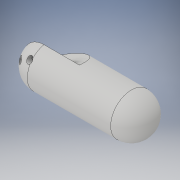
# Autodesk Inventor part: P1704_003_mainGauche
Saved by Autodesk Inventor 2019 (Build 230136000, 136)
## iProperties
Created: 2019-04-29
Part Number: P1704_003_mainGauche
Material: Générique
Document SubType Name: Modeling
Designer: Joan.MAILLARD
Density: 1 g/cm^3
Appearance: Par défaut
Author: Joan.MAILLARD
Autodesk Inventor part; units mm, degrees
ref_plane "YZ Plane" through (0, 0, 0) normal (1, 0, 0) x (0, 1, 0)
ref_plane "XZ Plane" through (0, 0, 0) normal (0, 1, 0) x (-1, 0, 0)
sketch "Esquisse1" plane through (0, 0, 0) normal (0, 1, 0) x (-1, 0, 0)
  line L0 (0, 0) -> (-100, 0)
  line L1 (-100, 0) -> (-100, -25)
  line L2 (-100, -25) -> (0, -25)
  line L3 (0, -25) -> (0, 0)
  arc A0 (0, -25) -> (25, 0) centre (0, 0) ccw
  line L4 (25, 0) -> (0, 0)
  line L5 (0, 0) -> (0, -25)
  line L6 (-100, 0) -> (-100, -25)
  arc A1 (-125, 0) -> (-100, -25) centre (-100, 0) ccw
  line L7 (-100, 0) -> (-125, 0)
  dimension "d1" = 25
  dimension "d2" = 100
  constraints: 16 end point, 4 line through centre, 4 point on circle, 3 equal length, 2 centre point, 2 coincident, 2 horizontal, 2 perpendicular, 1 vertical
  measures "d1" distance of L2.end L0.start
  measures "d2" distance of L1.end L2.end
revolve "Révolution1" add sketch "Esquisse1" angle 360 about axis through (0, 0, 0) along (1, 0, 0)
ref_plane "Plan de construction1" through (50, 0, -25) normal (0, 0, 1) x (1, 0, 0)
sketch "Esquisse2" plane through (50, 0, -25) normal (0, 0, 1) x (1, 0, 0)
  arc A0 (-50, 25) -> (-50, -25) centre (-50, 0) ccw projected
  line L0 (-50, 0) -> (-71.6506, -12.5)
  line L1 (-71.6506, -12.5) -> (-84.1506, 9.1506)
  line L2 (-84.1506, 9.1506) -> (-62.5, 21.6506)
  line L3 (-62.5, 21.6506) -> (-50, 0)
  line L4 (-50, 0) -> (-31.3481, 0) construction
  line L5 (-50, 0) -> (-62.5, 21.6506)
  line L6 (-62.5, 21.6506) -> (-19.1987, 46.6506)
  line L7 (-19.1987, 46.6506) -> (-6.6987, 25)
  line L8 (-6.6987, 25) -> (-50, 0)
  line L9 (-50, -25) -> (-50, 25) construction
  line L10 (-50, 25) -> (75, 25) construction
  line L11 (-50, 25) -> (50, 25) construction
  dimension "d9" = 120
  constraints: 20 end point, 4 parallel, 3 perpendicular, 2 point on circle, 2 point on line, 1 horizontal
  measures "d9" angle of L4 L3
extrude "Extrusion1" cut sketch "Esquisse2" along normal blind 30
ref_plane "Plan de construction2" through (50, 0, 35) normal (0, 0, -1) x (-1, 0, 0)
sketch "Esquisse3" plane through (50, 0, 35) normal (0, 0, -1) x (-1, 0, 0)
  line L0 (50, 0) -> (71.2132, -12.2474) construction
  line L1 (71.2132, -12.2474) -> (50, 0) construction
  line L2 (50, 0) -> (50, 0) construction
  line L3 (65.2228, 7.3769) -> (52.2324, 14.8769) construction
  circle A0 centre (65.2228, 7.3769) radius 1.7
  circle A1 centre (52.2324, 14.8769) radius 1.7
  line L4 (71.2132, -12.2474) -> (93.5005, 26.3552) construction
  line L5 (52.2324, 14.8769) -> (45.2324, 2.7526) construction
  line L6 (6.6987, 25) -> (-50, 25) construction
  dimension "d12" = 14
  dimension "d22" = 3.4
  dimension "d23" = 3.4
  dimension "d30" = 15
  dimension "d31" = 30
  constraints: 8 end point, 2 centre point, 2 coincident, 2 perpendicular, 1 collinear, 1 parallel, 1 other
  measures "d12" distance from line of L0 L3.start
  measures "d22" diameter of A0
  measures "d23" diameter of A1
  measures "d30" distance from line of L4 A0.centre
  measures "d31" distance from line of L4 L5.start
extrude "Extrusion2" cut sketch "Esquisse3" along normal blind 30
sketch "Esquisse4" plane through (50, 0, 35) normal (0, 0, -1) x (-1, 0, 0)
  circle A0 centre (65.2228, 7.3769) radius 1.7 projected
  circle A1 centre (65.2228, 7.3769) radius 3.25
  circle A2 centre (52.2324, 14.8769) radius 1.7 projected
  circle A3 centre (52.2324, 14.8769) radius 3.25
  point P0 (50, 0)
  dimension "d26" = 6.5
  dimension "d27" = 6.5
  constraints: 2 centre point, 2 coincident
  measures "d26" diameter of A1
  measures "d27" diameter of A3
extrude "Extrusion3" cut sketch "Esquisse4" along normal blind 20
equation "\"d23\" = d22"
equation "\"d27\" = d26"
